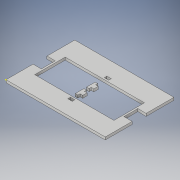
# Autodesk Inventor part: roof_v2
Saved by Autodesk Inventor 2017.2 (Build 212233000, 233)
## iProperties
Created: 2017-06-10
Part Number: roof_v2
Material: Generic
Document SubType Name: Modeling
Designer: SandeepSH
Density: 1 g/cm^3
Appearance: Default
Author: SandeepSH
Autodesk Inventor part; units mm, degrees
ref_plane "YZ Plane" through (0, 0, 0) normal (1, 0, 0) x (0, 1, 0)
ref_plane "XZ Plane" through (0, 0, 0) normal (0, 1, 0) x (-1, 0, 0)
ref_plane "XY Plane" through (0, 0, 0) normal (0, 0, 1) x (1, 0, 0)
sketch "Sketch1" plane through (0, 0, 0) normal (0, 1, 0) x (-1, 0, 0)
  line L0 (0, 0) -> (-114, 0)
  line L1 (-114, 0) -> (-114, -79)
  line L2 (-114, -79) -> (0, -79)
  line L3 (0, -79) -> (0, 0)
  dimension "d0" = 114
  dimension "d1" = 79
  constraints: 8 end point, 2 parallel, 1 horizontal, 1 perpendicular
  measures "d0" distance of L2.end L1.end
  measures "d1" distance of L1.end L0.end
extrude "Extrusion1" add sketch "Sketch1" along normal blind 3
sketch "Sketch2" plane through (0, 3, 0) normal (0, 1, 0) x (1, 0, 0)
  line L0 (0, 79) -> (0, 0) projected
  line L1 (0, 47) -> (9.5, 47)
  line L2 (9.5, 47) -> (9.5, 31)
  line L3 (9.5, 31) -> (0, 31)
  line L4 (0, 31) -> (0, 47)
  line L5 (114, 79) -> (0, 79) projected
  line L6 (57, 59.7224) -> (57, 18.4065)
  line L7 (114, 47) -> (104.5, 47)
  line L8 (104.5, 47) -> (104.5, 31)
  line L9 (104.5, 31) -> (114, 31)
  line L10 (114, 31) -> (114, 47)
  point P0 (9.5, 39)
  point P1 (104.5, 39)
  dimension "d4" = 9.5
  dimension "d5" = 16
  dimension "d6" = 8
  dimension "d7" = 40
  dimension "d8" = 57
  constraints: 18 end point, 5 symmetric about line, 2 midpoint, 2 parallel, 1 horizontal, 1 perpendicular, 1 point on line, 1 vertical
  measures "d4" distance of L2.end L3.end
  measures "d5" distance of L1.end L2.end
  measures "d6" distance from line of L1 point (9.5, 39)
  measures "d7" distance from line of L5 point (9.5, 39)
  measures "d8" distance between parallel lines of L0 L6
extrude "Extrusion2" cut sketch "Sketch2" against normal through all
sketch "Sketch3" plane through (0, 3, 0) normal (0, 1, 0) x (1, 0, 0)
  point P0 (0, 0)
sketch "Sketch4" plane through (0, 3, 0) normal (0, 1, 0) x (1, 0, 0)
  line L0 (9.5, 19.5) -> (104.5, 19.5)
  line L1 (104.5, 19.5) -> (104.5, 58.5)
  line L2 (104.5, 58.5) -> (9.5, 58.5)
  line L3 (9.5, 58.5) -> (9.5, 19.5)
  line L4 (114, 79) -> (0, 79) projected
  line L5 (11.5, 21.5) -> (102.5, 21.5)
  line L6 (102.5, 21.5) -> (102.5, 56.5)
  line L7 (102.5, 56.5) -> (11.5, 56.5)
  line L8 (11.5, 56.5) -> (11.5, 21.5)
  point P0 (0, 0)
  point P1 (17.7335, 39)
  point P2 (97.752, 39)
  point P3 (11.5, 39)
  point P4 (57, 21.5)
  dimension "d11" = 95
  dimension "d12" = 39
  dimension "d13" = 40
  dimension "d14" = 19.5
  dimension "d15" = 40
  dimension "d16" = 91
  dimension "d17" = 35
  dimension "d18" = 17.5
  dimension "d19" = 40
  dimension "d20" = 47.5
  constraints: 16 end point, 4 parallel, 2 horizontal, 2 midpoint, 2 perpendicular
  measures "d11" distance of L2.end L1.end
  measures "d12" distance of L1.end L0.end
  measures "d13" distance from line of L4 point (17.733, 39)
  measures "d14" distance from line of L2 point (97.752, 39)
  measures "d15" distance from line of L4 point (97.752, 39)
  measures "d16" distance of L7.end L6.end
  measures "d17" distance of L6.end L5.end
  measures "d18" distance from line of L7 point (11.5, 39)
  measures "d19" distance from line of L4 point (11.5, 39)
  measures "d20" distance from line of L1 point (57, 21.5)
extrude "Extrusion3" cut sketch "Sketch4" against normal through all contours L8 L7 L6 L5
sketch "Sketch5" plane through (0, 3, 0) normal (0, 1, 0) x (1, 0, 0)
  line L0 (59.5, 19.5) -> (54.5, 19.5)
  line L1 (54.5, 19.5) -> (54.5, 16.5)
  line L2 (54.5, 16.5) -> (59.5, 16.5)
  line L3 (59.5, 16.5) -> (59.5, 19.5)
  line L4 (59.5, 19.5) -> (54.5, 16.5) construction
  line L5 (54.5, 19.5) -> (59.5, 16.5) construction
  line L6 (9.5, 19.5) -> (104.5, 19.5) projected
  line L7 (59.5, 58.5) -> (54.5, 58.5)
  line L8 (54.5, 58.5) -> (54.5, 61.5)
  line L9 (54.5, 61.5) -> (59.5, 61.5)
  line L10 (59.5, 61.5) -> (59.5, 58.5)
  line L11 (59.5, 58.5) -> (54.5, 61.5) construction
  line L12 (54.5, 58.5) -> (59.5, 61.5) construction
  line L13 (104.5, 58.5) -> (9.5, 58.5) projected
  point P0 (0, 0)
  point P1 (57, 18)
  point P2 (57, 60)
  dimension "d23" = 5
  dimension "d24" = 3
  dimension "d25" = 5
  dimension "d26" = 3
  constraints: 24 end point, 4 midpoint, 4 parallel, 2 collinear, 2 horizontal, 2 perpendicular
  measures "d23" distance of L2.end L1.end
  measures "d24" distance of L1.end L0.end
  measures "d25" distance of L8.end L9.end
  measures "d26" distance of L7.end L8.end
extrude "Extrusion4" cut sketch "Sketch5" against normal through all
sketch "Sketch6" plane through (0, 3, 0) normal (0, 1, 0) x (1, 0, 0)
  line L0 (59.5895, 38.8648) -> (53.5895, 38.8648)
  line L1 (53.5895, 38.8648) -> (53.5895, 48.8648)
  line L2 (53.5895, 48.8648) -> (59.5895, 48.8648)
  line L3 (59.5895, 48.8648) -> (59.5895, 38.8648)
  line L4 (59.5895, 38.8648) -> (56.5895, 38.8648)
  line L5 (56.5895, 38.8648) -> (56.5895, 41.3648)
  line L6 (56.5895, 41.3648) -> (59.5895, 41.3648)
  line L7 (59.5895, 41.3648) -> (59.5895, 38.8648)
  line L8 (59.5895, 48.8648) -> (56.5895, 48.8648)
  line L9 (56.5895, 48.8648) -> (56.5895, 46.3648)
  line L10 (56.5895, 46.3648) -> (59.5895, 46.3648)
  line L11 (59.5895, 46.3648) -> (59.5895, 48.8648)
  line L12 (59.5895, 25.9829) -> (53.5895, 25.9829)
  line L13 (53.5895, 25.9829) -> (53.5895, 35.9829)
  line L14 (53.5895, 35.9829) -> (59.5895, 35.9829)
  line L15 (59.5895, 35.9829) -> (59.5895, 25.9829)
  line L16 (59.5895, 25.9829) -> (56.5895, 25.9829)
  line L17 (56.5895, 25.9829) -> (56.5895, 28.4829)
  line L18 (56.5895, 28.4829) -> (59.5895, 28.4829)
  line L19 (59.5895, 28.4829) -> (59.5895, 25.9829)
  line L20 (59.5895, 35.9829) -> (56.5895, 35.9829)
  line L21 (56.5895, 35.9829) -> (56.5895, 33.4829)
  line L22 (56.5895, 33.4829) -> (59.5895, 33.4829)
  line L23 (59.5895, 33.4829) -> (59.5895, 35.9829)
  point P0 (0, 0)
  dimension "d29" = 6
  dimension "d30" = 10
  dimension "d31" = 3
  dimension "d32" = 2.5
  dimension "d33" = 3
  dimension "d34" = 2.5
  dimension "d35" = 6
  dimension "d36" = 10
  dimension "d37" = 3
  dimension "d38" = 2.5
  dimension "d39" = 3
  dimension "d40" = 2.5
  constraints: 48 end point, 12 parallel, 6 horizontal, 6 perpendicular
  measures "d29" distance of L1.end L2.end
  measures "d30" distance of L0.end L1.end
  measures "d31" distance of L5.end L6.end
  measures "d32" distance of L4.end L5.end
  measures "d33" distance of L10.end L9.end
  measures "d34" distance of L9.end L8.end
  measures "d35" distance of L13.end L14.end
  measures "d36" distance of L12.end L13.end
  measures "d37" distance of L17.end L18.end
  measures "d38" distance of L16.end L17.end
  measures "d39" distance of L22.end L21.end
  measures "d40" distance of L21.end L20.end
extrude "Extrusion5" add sketch "Sketch6" against normal blind 3 contours L0 L1 L2 L9 L10 L3 L6 L5 | L12 L13 L14 L21 L22 L15 L18 L17
equation "\"d6\" = 0.5 * d5"
equation "\"d14\" = 0.5 * d12"
equation "\"d15\" = d13"
equation "\"d18\" = 0.5 * d17"
equation "\"d19\" = d13"
equation "\"d20\" = 0.5 * d11"
body "Solid1"
